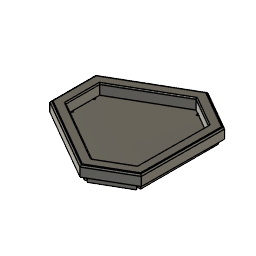
lid (Autodesk Fusion 360 design; units mm, degrees)
part number: 2026-07-20-10-30-57-472
Autodesk Fusion 360 part; units mm, degrees
sketch "Sketch1" plane through (0, 0, 0) normal (0, 0, 1) x (1, 0, 0)
  line L0 (-55.409, -19.9711) -> (10.409, -57.9711)
  line L1 (-48.8655, -12.202) -> (-47.8655, -10.4699)
  line L2 (26.9416, -50.2057) -> (44.2412, -40.2178)
  line L3 (-48.8655, 12.202) -> (-47.8655, 10.4699)
  line L4 (10.409, 57.9711) -> (8.6769, 56.9711)
  line L5 (33, 36.2178) -> (33, 40.2178)
  line L6 (10.409, -57.9711) -> (8.6769, -56.9711)
  line L7 (45, 38) -> (45, 36)
  line L8 (-56.9502, 0) -> (-56.9502, 18.2051)
  line L9 (14.8655, -46.6877) -> (18.3296, -48.6877)
  line L10 (-55.409, -19.9711) -> (-53.6769, -20.9711)
  line L11 (-47.8655, -10.4699) -> (-51.3296, -8.4699)
  line L12 (45, -38) -> (45, 38)
  line L13 (13.8655, -48.4198) -> (14.8655, -46.6877)
  line L14 (-55.409, 19.9711) -> (-50.409, 11.3109)
  line L15 (15.409, 49.3109) -> (10.409, 57.9711)
  line L16 (-55.409, 19.9711) -> (-53.6769, 20.9711)
  line L17 (10.409, 57.9711) -> (-55.409, 19.9711)
  line L18 (-50.409, -11.3109) -> (-55.409, -19.9711)
  line L19 (13.8655, 48.4198) -> (14.8655, 46.6877)
  line L20 (10.409, -57.9711) -> (15.409, -49.3109)
  line L21 (26.9416, -50.2057) -> (12.709, -58.4229)
  line L22 (35, 36.2178) -> (33, 36.2178)
  line L23 (45, -38) -> (45, -36)
  line L24 (-47.8655, 10.4699) -> (-51.3296, 8.4699)
  line L25 (-56.9502, 0) -> (-56.9502, -18.2051)
  line L26 (35, -38) -> (45, -38)
  line L27 (45, 36) -> (50.1191, 36) construction
  line L28 (35, -36.2178) -> (33, -36.2178)
  line L29 (33, -36.2178) -> (33, -40.2178)
  line L30 (14.8655, 46.6877) -> (18.3296, 48.6877)
  line L31 (-56.9502, 18.2051) -> (-51.3296, 8.4699)
  line L32 (-56.9502, 18.2051) -> (-51.3296, 8.4699)
  line L33 (18.3296, 48.6877) -> (12.709, 58.4229)
  line L34 (18.3296, -48.6877) -> (12.709, -58.4229)
  line L35 (13.8655, -48.4198) -> (15.409, -49.3109)
  line L36 (-50.409, 11.3109) -> (-48.8655, 12.202)
  line L37 (13.8655, 48.4198) -> (15.409, 49.3109)
  line L38 (35, 38) -> (35, 36.2178)
  line L39 (35, -36.2178) -> (35, -38)
  line L40 (33, -40.2178) -> (44.2412, -40.2178)
  line L41 (33, 40.2178) -> (44.2412, 40.2178)
  line L42 (35, 38) -> (45, 38)
  line L43 (12.709, 58.4229) -> (44.2412, 40.2178)
  line L44 (-50.409, -11.3109) -> (-48.8655, -12.202)
  line L45 (-51.3296, -8.4699) -> (-56.9502, -18.2051)
  line L46 (-47.6606, 10.415) -> (-51.2546, 8.34)
  line L47 (-48.8106, 12.4069) -> (-47.6606, 10.415)
  line L48 (-50.3541, 11.5158) -> (-48.8106, 12.4069)
  line L49 (-55.2041, 19.9162) -> (-50.3541, 11.5158)
  line L50 (10.3541, 57.7662) -> (-55.2041, 19.9162)
  line L51 (15.2041, 49.3658) -> (10.3541, 57.7662)
  line L52 (13.6606, 48.4747) -> (15.2041, 49.3658)
  line L53 (13.6606, 48.4747) -> (14.8106, 46.4828)
  line L54 (14.8106, 46.4828) -> (18.5345, 48.6328)
  line L55 (18.5345, 48.6328) -> (13.1188, 58.0131)
  line L56 (13.1188, 58.0131) -> (43.6814, 40.3678)
  line L57 (32.85, 40.3678) -> (43.6814, 40.3678)
  line L58 (32.85, 36.0678) -> (32.85, 40.3678)
  line L59 (35.15, 36.0678) -> (32.85, 36.0678)
  line L60 (35.15, 37.85) -> (35.15, 36.0678)
  line L61 (35.15, 37.85) -> (44.85, 37.85)
  line L62 (44.85, -37.85) -> (44.85, 37.85)
  line L63 (35.15, -37.85) -> (44.85, -37.85)
  line L64 (35.15, -36.0678) -> (35.15, -37.85)
  line L65 (35.15, -36.0678) -> (32.85, -36.0678)
  line L66 (32.85, -36.0678) -> (32.85, -40.3678)
  line L67 (32.85, -40.3678) -> (43.6814, -40.3678)
  line L68 (26.8666, -50.0758) -> (43.6814, -40.3678)
  line L69 (26.8666, -50.0758) -> (13.1188, -58.0131)
  line L70 (18.5345, -48.6328) -> (13.1188, -58.0131)
  line L71 (14.8106, -46.4828) -> (18.5345, -48.6328)
  line L72 (13.6606, -48.4747) -> (14.8106, -46.4828)
  line L73 (13.6606, -48.4747) -> (15.2041, -49.3658)
  line L74 (10.3541, -57.7662) -> (15.2041, -49.3658)
  line L75 (-55.2041, -19.9162) -> (10.3541, -57.7662)
  line L76 (-50.3541, -11.5158) -> (-55.2041, -19.9162)
  line L77 (-50.3541, -11.5158) -> (-48.8106, -12.4069)
  line L78 (-48.8106, -12.4069) -> (-47.6606, -10.415)
  line L79 (-47.6606, -10.415) -> (-51.3845, -8.265)
  line L80 (-51.3845, -8.265) -> (-56.8002, -17.6453)
  line L81 (-56.8002, 0) -> (-56.8002, -17.6453)
  line L82 (-51.4595, 8.3949) -> (-51.3845, 8.265)
  line L83 (-51.3845, 8.265) -> (-51.2546, 8.34)
  line L84 (-51.4595, 8.3949) -> (-56.8002, 17.6453)
  line L85 (-56.8002, 17.6453) -> (-56.8002, 0)
  point P0 (40, 0)
  point P1 (-20, -34.641)
  dimension "d27" = 47.8655
  dimension "d28" = 4
  dimension "d29" = 2
  dimension "d30" = 12
  dimension "d31" = 12
  dimension "d32" = 2
  dimension "d33" = 89.9502
  dimension "d34" = 1.7822
  dimension "d35" = 87.8655
  dimension "d36" = 27.8655
  dimension "d37" = 9.0847
  dimension "d38" = 92.8655
  dimension "d39" = 29.7478
  dimension "d40" = 27.5301
  dimension "d41" = 25.7478
  dimension "d42" = 46.4699
  dimension "d43" = 46.6877
  dimension "d44" = 48.4699
  dimension "d45" = 50.6877
  dimension "d46" = 30
  dimension "d47" = 78.2178
  dimension "d48" = 76.4356
  dimension "d49" = 80.4356
  dimension "d50" = 11.2412
  dimension "d51" = 76.4356
  dimension "d52" = 101.9502
  dimension "d53" = 10
  dimension "d54" = 101.9502
  dimension "d55" = 4
  dimension "d56" = 76.4356
  dimension "d57" = 80.8655
  dimension "d58" = 30
  dimension "d59" = 2
  dimension "d60" = 2
  dimension "d61" = 24.1711
  dimension "d62" = 5.1191
  dimension "d63" = 16.4344
  dimension "d64" = -0.15
  dimension "d66" = 50.0758
  dimension "d67" = 0.15
  constraint horizontal L26
  constraint perpendicular L12 L26
  constraint perpendicular L23 L26
  constraint horizontal L27
  constraint perpendicular L28 L29
  constraint parallel L2 L21
  constraint horizontal L8.start origin
  constraint perpendicular L24 L31
  constraint perpendicular L30 L33
  constraint perpendicular L9 L34
  constraint perpendicular L20 L35
  constraint perpendicular L3 L36
  constraint perpendicular L15 L37
  constraint perpendicular L22 L38
  constraint perpendicular L26 L39
  constraint perpendicular L29 L40
  constraint perpendicular L5 L41
  constraint perpendicular L7 L42
  constraint perpendicular L1 L44
  constraint perpendicular L10 L45
  constraint perpendicular L11 L45
  constraint collinear L9 L11
  constraint equal L1 L3
  constraint equal L1 L4
  constraint equal L1 L6
  constraint equal L1 L7
  constraint equal L1 L13
  constraint equal L1 L19
  constraint equal L1 L22
  constraint equal L1 L28
  constraint equal L5 L11
  constraint equal L35 L44
  constraint equal L31 L45
  constraint horizontal origin P0
  constraint perpendicular L3 L24
  constraint perpendicular L4 L15
  constraint collinear L4 L16
  constraint perpendicular L19 L30
  constraint perpendicular L19 L37
  constraint collinear L5 L29
  constraint equal L5 L24
  constraint equal L0 L17
  constraint equal L35 L36
  constraint equal L35 L37
  constraint equal L14 L18
  constraint equal L8 L25
  constraint equal L31 L33
  constraint perpendicular L46 L82
  constraint perpendicular L82 L83
  constraint parallel L31 L84
  constraint parallel L25 L85
  constraint coincident L24.end L31.end
  constraint horizontal L8.start L81.start
  constraint equal L82 L83
  constraint equal L81 L85
  measures "d27" horizontal distance of origin L1.end
  measures "d28" distance of L1 L45
  measures "d29" distance of L11 L44
  measures "d30" distance of L0 L11
  measures "d31" distance of L6 L11
  measures "d32" distance of L11 L35
  measures "d33" distance of L11 L43
  measures "d34" distance of L1 L18
  measures "d35" horizontal distance of P0 L1.end
  measures "d36" horizontal distance of P1 L1.end
  measures "d37" distance of L1.end L8
  measures "d38" distance of L1.end L12
  measures "d39" distance of L1.end L40
  measures "d40" distance of L1.end L26
  measures "d41" distance of L1.end L28
  measures "d42" distance of L1.end L27
  measures "d43" distance of L1.end L22
  measures "d44" distance of L1.end L42
  measures "d45" distance of L1.end L41
  measures "d46" angle of L25 L45
  measures "d47" distance of L20 L45
  measures "d48" distance of L13 L45
  measures "d49" distance of L34 L45
  measures "d50" distance of L21.end L9
  measures "d51" distance of L3 L33
  measures "d52" distance of L4 L21
  measures "d53" distance of L7 L38
  measures "d54" distance of L7 L25
  measures "d55" distance of L19 L33
  measures "d56" distance of L22 L40
  measures "d57" distance of L3.end L5
  measures "d58" angle of L33 L43
  measures "d59" distance of L23.end L26
  measures "d60" distance of L16.end L14
  measures "d61" vertical distance of P1 L1.end
  measures "d62" distance of L27.end L7
  measures "d63" distance of L2.start L21.end
  measures "d66" vertical distance of origin L68.start
  measures "d67" distance of L82.start L83
extrude "Extrude2" add sketch "Sketch1" against normal blind 5 contours L46 L47 L48 L49 L50 L51 L52 L53 L54 L55 L56 L57 L58 L59 L60 L61 L62 L63 L64 L65 L66 L67 L68 L69 L70 L71 L72 L73 L74 L75 L76 L77 L78 L79 L80 L81 L82 L83 L84 L85
sketch "Sketch2" plane through (0, 0, 0) normal (0, 0, 1) x (1, 0, 0)
  line L0 (10.3305, 62.1056) -> (-58.9502, 22.1063)
  line L1 (10.3305, 62.1056) -> (-58.9502, 22.1063)
  line L2 (-58.9502, -22.1063) -> (10.3305, -62.1056)
  line L3 (-58.9502, -22.1063) -> (10.3305, -62.1056)
  line L4 (-58.9502, 22.1063) -> (-58.9502, -22.1063)
  line L5 (10.3305, 62.1056) -> (48.6198, 39.9992)
  line L6 (48.6198, 39.9992) -> (48, -40.2178)
  line L7 (10.3305, -62.1056) -> (48, -40.2178)
  dimension "d92" = 48
  dimension "d93" = 107.57
  dimension "d94" = 119.557
  dimension "d95" = 119.841
  dimension "d96" = 107.57
  dimension "d97" = 79.9984
  dimension "d98" = 106.9502
  dimension "d99" = 40.2178
  constraint vertical L4
  constraint coincident L2.start L3.start
  constraint coincident L2.end L3.end
  constraint coincident L0.start L1.start
  constraint coincident L0.end L1.end
  constraint parallel L3 L5
  constraint equal L0 L2
  constraint equal L4 L5
  measures "d92" horizontal distance of origin L6.end
  measures "d93" distance of L5.end L4
  measures "d94" angle of L5 L6
  measures "d95" angle of L2 L7
  measures "d96" distance of L2 L5
  measures "d97" distance of L2.start L2.end
  measures "d98" distance of L6.end L4
  measures "d99" vertical distance of origin L6.end
extrude "Extrude3" add sketch "Sketch2" along normal blind 10 thin wall 10 inside
chamfer "Chamfer1" distance 1.5 angle 45 6 edges at (-24.3099, 42.1059, 10) (29.4751, 51.0524, 10) (48.3099, -0.1093, 10) (29.1652, -51.1617, 10) (-24.3099, -42.1059, 10) (-58.9502, 0, 10)
fillet "Fillet1" radius 1 6 edges at (-57.4502, 0, 10) (-23.5599, 40.8069, 10) (-23.5611, -40.8062, 10) (28.4174, -49.8614, 10) (46.8099, -0.1068, 10) (28.7218, 49.7553, 10)
fillet "Fillet2" radius 1 6 edges at (38.3097, -0.0927, 10) (24.1794, -42.4931, 10) (-19.3179, -33.4411, 10) (-48.9502, 0, 10) (-19.3099, 33.4457, 10) (24.4528, 42.405, 10)
